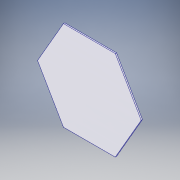
# Autodesk Inventor part: Frosted Top v1
Saved by Autodesk Inventor 2019 (Build 230136000, 136)
## iProperties
Created: 2021-07-14
Part Number: Frosted Top v1
Material: Generic
Document SubType Name: Modeling
Designer: Lix
Density: 1 g/cm^3
Appearance: Cool White
Author: Lix
Autodesk Inventor part; units mm, degrees
ref_plane "YZ Plane" through (0, 0, 0) normal (1, 0, 0) x (0, 1, 0)
ref_plane "XZ Plane" through (0, 0, 0) normal (0, 1, 0) x (-1, 0, 0)
ref_plane "XY Plane" through (0, 0, 0) normal (0, 0, 1) x (1, 0, 0)
sketch "Sketch1" plane through (0, 0, 0) normal (0, 0, 1) x (1, 0, 0)
  line L0 (-40.9919, 71) -> (40.9919, 71)
  line L1 (40.9919, 71) -> (81.9837, 0)
  line L2 (81.9837, 0) -> (40.9919, -71)
  line L3 (40.9919, -71) -> (-40.9919, -71)
  line L4 (-40.9919, -71) -> (-81.9837, 0)
  line L5 (-81.9837, 0) -> (-40.9919, 71)
  point P0 (0, 0)
  point P1 (0, 0)
  dimension "d0" = 142
  constraints: 12 end point, 1 coincident, 1 horizontal, 13 other
  measures "d0" distance between parallel lines of L4 L1
extrude "Extrusion1" add sketch "Sketch1" along normal blind 2
body "Solid1"
